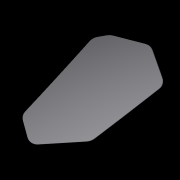
# Autodesk Inventor part: ShadeBasicRight
Saved by Autodesk Inventor 2020 (Build 240168000, 168)
## iProperties
Created: 2015-07-22
Part Number: ShadeBasicRight
Material: Generic
Document SubType Name: Modeling
Designer: Val
Density: 1 g/cm^3
Appearance: Default
Author: Val
Autodesk Inventor part; units mm, degrees
ref_plane "YZ Plane" through (0, 0, 0) normal (1, 0, 0) x (0, 1, 0)
ref_plane "XZ Plane" through (0, 0, 0) normal (0, 1, 0) x (-1, 0, 0)
ref_plane "XY Plane" through (0, 0, 0) normal (0, 0, 1) x (1, 0, 0)
sketch "Base" plane through (0, 0, 0) normal (0, 0, 1) x (1, 0, 0)
  line L0 (11.024, 19.2429) -> (25.9786, 10.3086)
  line L1 (25.9786, 10.3086) -> (26.9269, -6.9521)
  line L2 (26.9269, -6.9521) -> (-9.2224, -20.9335)
  line L3 (-9.2224, -20.9335) -> (-33.9554, -15.2892)
  line L4 (-33.9554, -15.2892) -> (-33.7656, -2.5777)
  line L5 (-33.7656, -2.5777) -> (3.7833, 20.1134)
  line L6 (3.7833, 20.1134) -> (11.024, 19.2429)
  circle A0 centre (-6.3323, 4.8408) radius 2.5
  circle A1 centre (-11.8617, -1.6151) radius 2.5
  line L7 (-6.3323, 4.8408) -> (-11.8617, -1.6151) construction
  line L8 (2.9132, 5.1838) -> (6.4665, -2.5379) construction
  circle A2 centre (2.9132, 5.1838) radius 2.5
  circle A3 centre (6.4665, -2.5379) radius 2.5
  line L9 (-8.3083, -9.3368) -> (0.1918, -9.3368) construction
  circle A4 centre (0.1918, -9.3368) radius 2.5
  circle A5 centre (-8.3083, -9.3368) radius 2.5
  line L10 (0.6421, 4.1388) -> (4.1954, -3.583)
  line L11 (5.1843, 6.2289) -> (8.7376, -1.4928)
  line L12 (-8.2311, 6.4671) -> (-13.7604, 0.0112)
  line L13 (-4.4336, 3.2146) -> (-9.9629, -3.2413)
  line L14 (-8.3083, -6.8368) -> (0.1918, -6.8368)
  line L15 (-8.3083, -11.8368) -> (0.1918, -11.8368)
  line L16 (-11.8617, -1.6151) -> (-18.4752, -9.3368) construction
  line L17 (-18.4752, -9.3368) -> (-8.3083, -9.3368) construction
  line L18 (-11.8617, -1.6151) -> (-8.3083, -9.3368) construction
  line L19 (-18.4752, -9.3368) -> (4.6899, 1.323) construction
  point P0 (0, 0)
  point P1 (-9.097, 1.6129)
  point P2 (-4.0583, -9.3368)
  dimension "d8" = 146
  dimension "d12" = 108
  dimension "d13" = 124
  dimension "d14" = 156
  dimension "d15" = 142
  dimension "d16" = 122
  dimension "d17" = 59.934
  dimension "d20" = 5
  dimension "d62" = 25.5
  constraints: 40 end point, 12 point on circle, 12 tangent, 6 centre point, 4 coincident, 4 equal radius, 3 equal length, 3 midpoint, 2 collinear, 2 horizontal, 1 parallel, 4 other
  measures "d8" angle of L2 L3
  measures "d12" angle of L1 L2
  measures "d13" angle of L1 L0
  measures "d14" angle of L0 L6
  measures "d15" angle of L6 L5
  measures "d16" angle of L4 L5
  measures "d17" horizontal distance of L0.end L3.end
  measures "d20" diameter of A0
  measures "d62" distance of L16.end L19.end
extrude "BaseFeature" add sketch "Base" along normal mid plane 14 contours L0 L1 L2 L3 L4 L5 L6 | A0 | A0 L13 A1 L12 | A1 | A2 | A2 L11 A3 L10 | A3 | A4 | A4 L15 A5 L14 | A5
fillet "SmallFilletsFeature" radius 4 4 edges at (-33.7656, -2.5777, 0) (-33.9554, -15.2892, 0) (26.9269, -6.9521, 0) (25.9786, 10.3086, 0)
fillet "LargeFilletsFeature" radius 6 3 edges at (-9.2224, -20.9335, 0) (3.7833, 20.1134, 0) (11.024, 19.2429, 0)
ref_plane "SlopeProfileMiddlePlane" through (-8.6558, -2.3082, 0) normal (0.0635705, -0.9979774, 0) x (0, 0, 1)
ref_plane "SlopeProfilePlane" through (-7.5115, -20.2717, 0) normal (0.0635705, -0.9979774, 0) x (0, 0, 1)
sketch "SlopeProfileIntersect" plane through (-8.6558, -2.3082, 0) normal (0.0635705, -0.9979774, 0) x (0, 0, 1)
  arc A0 (7, -8.785) -> (-59.3577, 91.215) centre (-101.5281, -8.785) ccw
  arc A1 (-59.3577, -108.785) -> (7, -8.785) centre (-101.5281, -8.785) ccw
  line L0 (-59.3577, 91.215) -> (-59.3577, -108.785)
  line L1 (-128.2497, -8.785) -> (44.802, -8.785) construction
  line L2 (7, -12.0068) -> (7, 23.1095) construction
  point P0 (0, -8.785)
  point P1 (-59.3577, -8.785)
  dimension "d72" = 66.3577
  dimension "d84" = 200
  constraints: 5 point on line, 4 point on circle, 2 centre point, 2 end point, 1 concentric, 1 midpoint, 1 vertical
  measures "d72" distance from line of L0 A0.start
  measures "d84" distance of L0.start L0.end
revolve "SlopeProfileIntersectFeature" cut sketch "SlopeProfileIntersect" angle 360 about axis through (-99.6863, -8.1067, -59.3577) along (0.9979774, 0.0635705, 0) keep common part
sketch "SlopeProfileSubtract" plane through (-8.6558, -2.3082, 0) normal (0.0635705, -0.9979774, 0) x (0, 0, 1)
  arc A0 (7, -8.785) -> (-59.3577, 91.215) centre (-101.5281, -8.785) ccw construction
  arc A1 (-59.3577, -108.785) -> (7, -8.785) centre (-101.5281, -8.785) ccw construction
  arc A2 (2.9991, -8.3402) -> (-59.3577, 86.859) centre (-101.5281, -8.785) ccw
  arc A3 (-59.3577, -104.429) -> (2.9991, -8.3402) centre (-101.5281, -8.785) ccw
  line L0 (-59.3577, 86.859) -> (-59.3577, -104.429)
  line L1 (-128.2497, -8.785) -> (44.802, -8.785) construction
  line L2 (-59.3577, 86.859) -> (-59.3577, 91.215) construction
  point P0 (0, -8.785)
  point P1 (-59.3577, -8.785)
  dimension "d70" = 4
  constraints: 4 end point, 4 point on circle, 2 centre point, 1 midpoint, 1 perpendicular, 1 point on line, 1 vertical, 1 other
  measures "d70" radial gap between concentric circles of A0 A2
revolve "SlopeProfileSubtractFeature" cut sketch "SlopeProfileSubtract" angle 360 about axis through (-95.3391, -7.8298, -59.3577) along (0.9979774, 0.0635705, 0)
mirror "Mirror1" about plane through (0, 0, 0) normal (1, 0, 0) remove original yes
body "Solid1"
